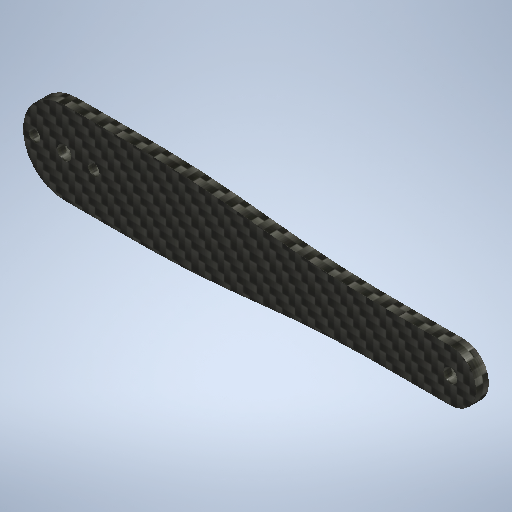
# Autodesk Inventor part: RT_ARM_MC_002
Saved by Autodesk Inventor 2025.4 (Build 294407000, 407)
## iProperties
Created: 2026-04-27
Part Number: RT_ARM_MC_002
Material: CFRP
Document SubType Name: Modeling
Designer: louis
Density: 1.43 g/cm^3
Appearance: Carbon Fiber 1
Author: louis
Autodesk Inventor part; units mm, degrees
ref_plane "YZ Plane" through (0, 0, 0) normal (1, 0, 0) x (0, 1, 0)
ref_plane "XZ Plane" through (0, 0, 0) normal (0, 1, 0) x (-1, 0, 0)
ref_plane "XY Plane" through (0, 0, 0) normal (0, 0, 1) x (1, 0, 0)
sketch "Sketch2" plane through (0, 0, 0) normal (0, 1, 0) x (-1, 0, 0)
  circle A0 centre (0, 0) radius 16
  circle A1 centre (-150, 0) radius 10
  line L0 (0, 0) -> (-150, 0)
  line L1 (0, 16) -> (-20, 16)
  line L2 (-150, 10) -> (-130, 10)
  spline S0 degree 4 poles (-20, 16) (-33.7807, 16) (-61.342, 16) (-88.658, 10) (-116.2193, 10) (-130, 10) knots 0 0 0 0 0 0.5 1 1 1 1 1
  line L3 (0, 0) -> (0, 16) construction
  line L4 (-150, 0) -> (-150, 10) construction
  line L5 (0, -16) -> (-20, -16)
  line L6 (-150, -10) -> (-130, -10)
  spline S1 degree 4 poles (-20, -16) (-33.7807, -16) (-61.342, -16) (-88.658, -10) (-116.2193, -10) (-130, -10) knots 0 0 0 0 0 0.5 1 1 1 1 1
  line L7 (11.5, 0) -> (-11.5, 0) construction
  dimension "d0" = 32
  dimension "d1" = 20
  dimension "d2" = 150
  dimension "d3" = 20
  dimension "d4" = 20
  dimension "d5" = 23
  constraints: 16 end point, 7 horizontal, 5 coincident, 4 symmetric about line, 2 vertical, 1 midpoint, 1 point on line, 10 other
  measures "d2" distance of L0.start L0.end
  measures "d3" distance of L1.start L1.end
  measures "d4" distance of L2.start L2.end
  measures "d5" distance of L7.start L7.end
extrude "Extrusion1" add sketch "Sketch2" along normal blind 5
hole "Hole1" at (-11.5, 0, 0) at (11.5, 0, 0) direction (0, 1, 0) diameter 4.5 end through all clearance for "Socket Head Cap Screw" size "M4" standard "Ansi Metric M Profile"
hole "Hole2" at (150, 0, 0) at (0, 0, 0) direction (0, 1, 0) diameter 5.5 end through all clearance for "Socket Head Cap Screw" size "M5" standard "Ansi Metric M Profile"
body "Solid1"
